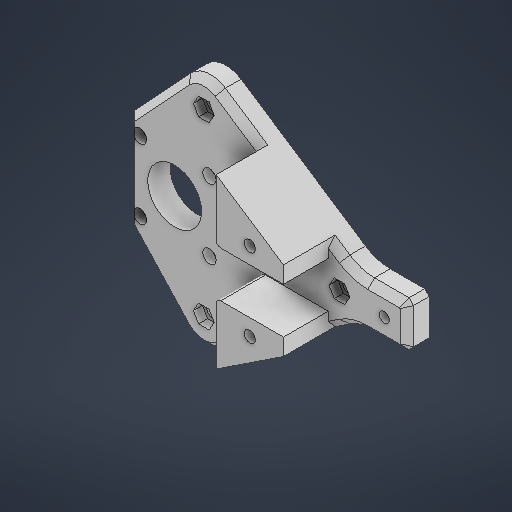
# Autodesk Inventor part: y axis motor holder
Saved by Autodesk Inventor 2026 (Build 300175000, 175)
## iProperties
Created: 2025-02-02
Part Number: y axis motor holder
Material: Generic
Document SubType Name: Modeling
Designer: jerem
Density: 1 g/cm^3
Appearance: Default
Author: jerem
## iProperties of the stored document y axis motor holder_3DPrint.ipt
Created: 2025-02-21
Part Number: y axis motor holder_3DPrint
Material: Generic
Document SubType Name: Modeling
Designer: jerem
Density: 1 g/cm^3
Appearance: Default
Author: jerem
Autodesk Inventor part; units mm, degrees
ref_plane "YZ Plane" through (0, 0, 0) normal (1, 0, 0) x (0, 1, 0)
ref_plane "XZ Plane" through (0, 0, 0) normal (0, 1, 0) x (-1, 0, 0)
ref_plane "XY Plane" through (0, 0, 0) normal (0, 0, 1) x (1, 0, 0)
sketch "Sketch1" plane through (0, 0, 0) normal (0, 0, 1) x (1, 0, 0)
  line L0 (0, 0) -> (30.25, 0) construction
  line L1 (0, 0) -> (-30.25, 0) construction
  line L2 (-30.25, 0) -> (-30.25, 40) construction
  line L3 (-30.25, 0) -> (-30.25, -40) construction
  circle A0 centre (-30.25, 40) radius 2.7
  circle A1 centre (-30.25, -40) radius 2.7
  circle A2 centre (30.25, 0) radius 2.7
  circle A3 centre (-30.25, 40) radius 12
  circle A4 centre (-30.25, -40) radius 12
  circle A5 centre (30.25, 0) radius 12
  line L4 (36.868172, -10.009985) -> (-23.631828, -50.009985)
  line L5 (-42.25, 40) -> (-42.25, -40)
  line L6 (-23.631828, 50.009985) -> (36.868172, 10.009985)
  line L7 (30.25, 0) -> (50.25, 0) construction
  circle A6 centre (50.25, 0) radius 10
  circle A7 centre (50.25, 0) radius 2.25
  line L8 (50.25746, 9.999997) -> (36.868172, 10.009985)
  line L9 (50.25746, -9.999997) -> (36.868172, -10.009985)
  line L10 (-27.75, -15.5) -> (-58.75, -15.5) construction
  line L11 (-58.75, -15.5) -> (-58.75, 15.5) construction
  line L12 (-58.75, 15.5) -> (-27.75, 15.5) construction
  line L13 (-27.75, 15.5) -> (-27.75, -15.5) construction
  line L14 (-27.75, -15.5) -> (-58.75, 15.5) construction
  line L15 (-58.75, -15.5) -> (-27.75, 15.5) construction
  line L16 (-22.25, -21) -> (-64.25, -21) construction
  line L17 (-64.25, -21) -> (-64.25, 21)
  line L18 (-64.25, 21) -> (-22.25, 21) construction
  line L19 (-22.25, 21) -> (-22.25, -21) construction
  line L20 (-22.25, -21) -> (-64.25, 21) construction
  line L21 (-64.25, -21) -> (-22.25, 21) construction
  line L22 (-43.25, 0) -> (-42.25, 0) construction
  circle A8 centre (-27.75, 15.5) radius 2
  circle A9 centre (-58.75, 15.5) radius 2
  circle A10 centre (-58.75, -15.5) radius 2
  circle A11 centre (-27.75, -15.5) radius 2
  line L23 (-64.25, 21) -> (-39.046516, 48.162187)
  line L24 (-64.25, -21) -> (-39.046516, -48.162187)
  circle A12 centre (-43.25, 0) radius 12
  circle A13 centre (10.25, 0) radius 2.25
  line L25 (50.25746, 9.999997) -> (60.257457, 9.992538)
  line L26 (60.257457, 9.992538) -> (60.242549, -9.992549)
  line L27 (60.242549, -9.992549) -> (50.25746, -9.999997)
  point P0 (41.35, -4.559605)
  point P1 (41.35, 4.559605)
  point P2 (60.249997, -0.00746)
  dimension "d0" = 60.5
  dimension "d1" = 5.4
  dimension "d2" = 80
  dimension "d3" = 24
  dimension "d57" = 20
  dimension "d58" = 20
  dimension "d61" = 31
  dimension "d63" = 42
  dimension "d65" = 1
  dimension "d66" = 4
  dimension "d67" = 4
  dimension "d68" = 4
  dimension "d69" = 4
  dimension "d70" = 4.5
  dimension "d71" = 24
  dimension "d74" = 4.5
  dimension "d75" = 20
  constraints: 56 end point, 14 centre point, 13 coincident, 12 tangent, 10 point on circle, 6 horizontal, 5 midpoint, 4 equal length, 4 equal radius, 4 parallel, 4 perpendicular, 2 point on line, 2 vertical, 1 collinear
  measures "d0" distance of L0.end L1.end
  measures "d1" diameter of A0
  measures "d2" distance of L3.end L2.end
  measures "d3" diameter of A3
  measures "d57" distance of L7.start L7.end
  measures "d58" diameter of A6
  measures "d61" distance of L10.end L11.end
  measures "d63" distance of L16.end L17.end
  measures "d65" distance of L22.end L22.start
  measures "d66" diameter of A8
  measures "d67" diameter of A9
  measures "d68" diameter of A10
  measures "d69" diameter of A11
  measures "d70" diameter of A7
  measures "d71" diameter of A12
  measures "d74" diameter of A13
  measures "d75" distance of L0.end A13.centre
sketch "Sketch1 outline for Extrusion1" plane through (0, 0, 0) normal (0, 0, 1) x (1, 0, 0)
  arc A0 (-23.631828, 50.009985) -> (-39.046516, 48.162187) centre (-30.25, 40) ccw
  line L0 (-39.046516, 48.162187) -> (-64.25, 21)
  line L1 (-64.25, 21) -> (-64.25, -21)
  line L2 (-64.25, -21) -> (-39.046516, -48.162187)
  arc A1 (-39.046516, -48.162187) -> (-23.631828, -50.009985) centre (-30.25, -40) ccw
  line L3 (-23.631828, -50.009985) -> (36.868172, -10.009985)
  line L4 (36.868172, -10.009985) -> (60.242549, -9.992549)
  line L5 (60.242549, -9.992549) -> (60.257457, 9.992538)
  line L6 (60.257457, 9.992538) -> (36.868172, 10.009985)
  line L7 (36.868172, 10.009985) -> (-23.631828, 50.009985)
  circle A2 centre (-30.25, 40) radius 2.7
  circle A3 centre (10.25, 0) radius 2.25
  circle A4 centre (-27.75, 15.5) radius 2
  circle A5 centre (-58.75, -15.5) radius 2
  circle A6 centre (-27.75, -15.5) radius 2
  circle A7 centre (-43.25, 0) radius 12
  circle A8 centre (-58.75, 15.5) radius 2
  circle A9 centre (30.25, 0) radius 2.7
  circle A10 centre (-30.25, -40) radius 2.7
  circle A11 centre (50.25, 0) radius 2.25
extrude "Extrusion1" add sketch "Sketch1 outline for Extrusion1" against normal blind 10
fillet "Fillet1" radius 20 2 edges at (36.8682, 10.01, -5) (36.8682, -10.01, -5)
chamfer "Chamfer7" distance 2 angle 45 2 edges at (60.2575, 9.9925, -5) (60.2425, -9.9925, -5)
sketch "Sketch8" plane through (0, 0, 0) normal (0, 0, 1) x (1, 0, 0)
  line L0 (58.242549, -9.994041) -> (60.244041, -7.992549)
  line L1 (58.242549, -9.994041) -> (42.873828, -10.005505)
  arc A0 (42.873828, -10.005505) -> (31.85846, -13.322191) centre (42.888747, -30.0055) ccw
  line L2 (31.85846, -13.322191) -> (-23.631828, -50.009985)
  arc A1 (-39.046516, -48.162187) -> (-23.631828, -50.009985) centre (-30.25, -40) ccw
  line L3 (-39.046516, -48.162187) -> (-64.25, -21)
  line L4 (-64.25, -21) -> (-64.25, 21)
  line L5 (-64.25, 21) -> (-39.046516, 48.162187)
  arc A2 (-23.631828, 50.009985) -> (-39.046516, 48.162187) centre (-30.25, 40) ccw
  line L6 (-23.631828, 50.009985) -> (31.85846, 13.322191)
  arc A3 (31.85846, 13.322191) -> (42.873828, 10.005505) centre (42.888747, 30.0055) ccw
  line L7 (42.873828, 10.005505) -> (58.257457, 9.99403)
  line L8 (60.255965, 7.992538) -> (58.257457, 9.99403)
  line L9 (60.255965, 7.992538) -> (60.244041, -7.992549)
  circle A4 centre (30.25, 0) radius 2.7
  circle A5 centre (50.25, 0) radius 2.25
  circle A6 centre (-30.25, -40) radius 2.7
  circle A7 centre (-43.25, 0) radius 12
  circle A8 centre (-58.75, -15.5) radius 2
  circle A9 centre (-58.75, 15.5) radius 2
  circle A10 centre (10.25, 0) radius 2.25
  circle A11 centre (-27.75, 15.5) radius 2
  circle A12 centre (-27.75, -15.5) radius 2
  circle A13 centre (-30.25, 40) radius 2.7
  line L10 (-32.573835, 44.025) -> (-27.926165, 44.025)
  line L11 (-27.926165, 44.025) -> (-25.60233, 40)
  line L12 (-25.60233, 40) -> (-27.926165, 35.975)
  line L13 (-27.926165, 35.975) -> (-32.573835, 35.975)
  line L14 (-32.573835, 35.975) -> (-34.89767, 40)
  line L15 (-34.89767, 40) -> (-32.573835, 44.025)
  line L16 (27.926165, 4.025) -> (32.573835, 4.025)
  line L17 (32.573835, 4.025) -> (34.89767, 0)
  line L18 (34.89767, 0) -> (32.573835, -4.025)
  line L19 (32.573835, -4.025) -> (27.926165, -4.025)
  line L20 (27.926165, -4.025) -> (25.60233, 0)
  line L21 (25.60233, 0) -> (27.926165, 4.025)
  line L22 (-32.573835, -35.975) -> (-27.926165, -35.975)
  line L23 (-27.926165, -35.975) -> (-25.60233, -40)
  line L24 (-25.60233, -40) -> (-27.926165, -44.025)
  line L25 (-27.926165, -44.025) -> (-32.573835, -44.025)
  line L26 (-32.573835, -44.025) -> (-34.89767, -40)
  line L27 (-34.89767, -40) -> (-32.573835, -35.975)
  point P0 (0, 0)
  dimension "d97" = 8.05
  dimension "d98" = 8.05
  dimension "d99" = 8.05
  constraints: 36 end point, 3 coincident, 3 horizontal, 39 other
  measures "d97" distance between parallel lines of L13 L10
  measures "d98" distance between parallel lines of L19 L16
  measures "d99" distance between parallel lines of L25 L22
extrude "Extrusion9" cut sketch "Sketch8" against normal blind 4 contours L10 L11 L12 L13 L14 L15 | L16 L17 L18 L19 L20 L21 | L22 L23 L24 L25 L26 L27
sketch "Sketch5" plane through (0, 0, 0) normal (0, 0, 1) x (1, 0, 0)
  line L0 (42.873828, -10.005505) -> (58.242549, -9.994041)
  arc A0 (31.85846, 13.322191) -> (42.873828, 10.005505) centre (42.888747, 30.0055) ccw
  line L1 (31.85846, 13.322191) -> (-23.631828, 50.009985)
  arc A1 (-23.631828, 50.009985) -> (-39.046516, 48.162187) centre (-30.25, 40) ccw
  line L2 (-39.046516, 48.162187) -> (-64.25, 21)
  line L3 (-64.25, 21) -> (-64.25, -21)
  line L4 (-64.25, -21) -> (-39.046516, -48.162187)
  arc A2 (-39.046516, -48.162187) -> (-23.631828, -50.009985) centre (-30.25, -40) ccw
  line L5 (-23.631828, -50.009985) -> (31.85846, -13.322191)
  arc A3 (42.873828, -10.005505) -> (31.85846, -13.322191) centre (42.888747, -30.0055) ccw
  circle A4 centre (50.25, 0) radius 2.25
  circle A5 centre (-27.75, -15.5) radius 2
  circle A6 centre (-27.75, 15.5) radius 2
  circle A7 centre (-58.75, 15.5) radius 2
  circle A8 centre (-58.75, -15.5) radius 2
  circle A9 centre (-43.25, 0) radius 12
  line L6 (-4.75, -10.2) -> (-4.75, -37.526132)
  line L7 (25.25, -10.2) -> (25.25, -17.691421)
  line L8 (-4.75, -10.2) -> (25.25, -10.2)
  line L9 (60.244041, -7.992549) -> (60.255965, 7.992538)
  line L10 (58.257457, 9.99403) -> (42.873828, 10.005505)
  line L11 (60.244041, -7.992549) -> (58.242549, -9.994041)
  line L12 (58.257457, 9.99403) -> (60.255965, 7.992538)
  point P0 (0, 0)
  dimension "d92" = 30
  dimension "d93" = 10.2
  dimension "d106" = 25
  constraints: 6 end point, 2 point on line, 1 horizontal, 1 parallel, 1 vertical
  measures "d92" distance of L6.start L7.start
  measures "d93" distance from line of L8 point (0, 0)
  measures "d106" distance from line of A4.centre L7
extrude "Extrusion6" add sketch "Sketch5" along normal blind 20 contours L5 L6 L8 L7
sketch "Sketch9" plane through (0, 0, 20) normal (0, 0, 1) x (1, 0, 0)
  circle A0 centre (10.25, 0) radius 2.25
  line L0 (-4.75, -10.2) -> (-4.75, -37.526132)
  line L1 (-4.75, -37.526132) -> (25.25, -17.691421)
  line L2 (25.25, -17.691421) -> (25.25, -10.2)
  line L3 (25.25, -10.2) -> (-4.75, -10.2)
  line L4 (10.25, 0) -> (10.25, -17.5) construction
  circle A1 centre (10.25, -17.5) radius 2.5
  point P0 (0, 0)
  dimension "d102" = 17.5
  dimension "d103" = 5
  constraints: 2 end point, 1 centre point, 1 coincident, 1 vertical
  measures "d102" distance of L4.start L4.end
  measures "d103" diameter of A1
extrude "Extrusion10" cut sketch "Sketch9" against normal blind 5 contours A1
mirror "Mirror1" about plane through (0, 0, 0) normal (0, 1, 0) of "Extrusion6", "Extrusion10"
fillet "Fillet2" radius 2 2 edges at (-4.75, 10.2, 10) (-4.75, -10.2, 10)
sketch "Sketch10" plane through (0, 0, 0) normal (0, 0, 1) x (1, 0, 0)
  circle A0 centre (-58.75, 15.5) radius 2 projected
  circle A1 centre (-27.75, 15.5) radius 2 projected
  circle A2 centre (-27.75, -15.5) radius 2 projected
  circle A3 centre (-58.75, -15.5) radius 2 projected
  circle A4 centre (-58.75, -15.5) radius 3
  circle A5 centre (-27.75, -15.5) radius 3
  circle A6 centre (-27.75, 15.5) radius 3
  circle A7 centre (-58.75, 15.5) radius 3
  point P0 (0, 0)
  dimension "d108" = 6
  constraints: 4 centre point, 4 coincident, 3 equal radius
  measures "d108" diameter of A4
extrude "Extrusion11" cut sketch "Sketch10" against normal blind 4 contours A0 | A1 | A2 | A3 | A4 | A5 | A6 | A7
sketch "Sketch11" plane through (0, 0, -10) normal (0, 0, -1) x (-1, 0, 0)
  circle A0 centre (-50.25, 0) radius 2.25 projected
  circle A1 centre (-10.25, 0) radius 2.25 projected
  circle A2 centre (-50.25, 0) radius 4
  circle A3 centre (-10.25, 0) radius 4
  point P0 (0, 0)
  dimension "d111" = 8
  dimension "d112" = 8
  constraints: 2 centre point, 2 coincident
  measures "d111" diameter of A2
  measures "d112" diameter of A3
extrude "Extrusion12" cut sketch "Sketch11" against normal blind 5
chamfer "Chamfer8" distance 3 angle 45 16 edges at (-51.6483, 34.5811, 0) (-31.6782, 51.9147, 0) (-14.1909, 43.7681, 0) (-64.25, 0, 0) (-51.6483, -34.5811, 0) (-31.6782, -51.9147, 0) (-14.1909, -43.7681, 0) (37.1225, 10.8548, 0) (50.5656, 9.9998, 0) (28.5542, 15.5068, 0) (50.5582, -9.9998, 0) (37.1225, -10.8548, 0) (28.5542, -15.5068, 0) (60.25, 0, 0) (59.2567, 8.9933, 0) (59.2433, -8.9933, 0)
equation "\"b\" = 2"
body "Solid1"
